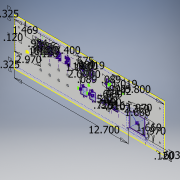
# Autodesk Inventor part: PDU_chassis
Saved by Autodesk Inventor 2017 (Build 210142000, 142)
## iProperties
Created: 2017-02-13
Part Number: PDU_chassis
Material: Generic
Document SubType Name: Modeling
Designer: Zara
Density: 1 g/cm^3
Appearance: Default
Author: Zara
Autodesk Inventor part; units mm, degrees
ref_plane "YZ Plane" through (0, 0, 0) normal (1, 0, 0) x (0, 1, 0)
ref_plane "XZ Plane" through (0, 0, 0) normal (0, 1, 0) x (-1, 0, 0)
ref_plane "XY Plane" through (0, 0, 0) normal (0, 0, 1) x (1, 0, 0)
sketch "Sketch1" plane through (0, 0, 0) normal (0, 0, 1) x (1, 0, 0)
  line L0 (-212.471, -66.294) -> (212.471, -66.294)
  line L1 (212.471, -66.294) -> (212.471, 66.294)
  line L2 (212.471, 66.294) -> (-212.471, 66.294)
  line L3 (-212.471, 66.294) -> (-212.471, -66.294)
  line L4 (-212.471, -66.294) -> (212.471, 66.294) construction
  line L5 (212.471, -66.294) -> (-212.471, 66.294) construction
  point P0 (0, 0)
  dimension "d0" = 424.942
  dimension "d1" = 132.588
  constraints: 12 end point, 2 midpoint, 2 parallel, 1 horizontal, 1 perpendicular
  measures "d0" distance of L1.end L2.end
  measures "d1" distance of L0.end L1.end
extrude "pdu" add sketch "Sketch1" along normal blind 1.651
sketch "dsub9 sketch" plane through (0, 0, 1.651) normal (0, 0, 1) x (1, 0, 0)
  line L0 (209.423, 58.039) -> (-209.423, 58.039) construction
  line L1 (-209.423, 58.039) -> (-209.423, -58.039) construction
  line L2 (-209.423, -58.039) -> (209.423, -58.039) construction
  line L3 (209.423, -58.039) -> (209.423, 58.039) construction
  line L4 (212.471, 66.294) -> (-212.471, 66.294) construction
  line L5 (-212.471, -66.294) -> (212.471, -66.294) construction
  line L6 (-212.471, 66.294) -> (-212.471, -66.294) construction
  line L7 (212.471, -66.294) -> (212.471, 66.294) construction
  arc A0 (-131.445, 36.9951) -> (-133.3231, 38.571) centre (-133.0452, 36.9951) ccw
  arc A1 (-133.3231, 19.3918) -> (-131.445, 20.9677) centre (-133.0452, 20.9677) ccw
  arc A2 (-142.621, 22.374) -> (-141.2987, 20.7981) centre (-141.0208, 22.374) ccw
  arc A3 (-141.2987, 37.1647) -> (-142.621, 35.5888) centre (-141.0208, 35.5888) ccw
  line L8 (-131.445, 36.9951) -> (-131.445, 20.9677)
  line L9 (-142.621, 35.5888) -> (-142.621, 22.374)
  line L10 (-141.2987, 37.1647) -> (-133.3231, 38.571)
  line L11 (-133.3231, 19.3918) -> (-141.2987, 20.7981)
  line L12 (-131.445, 28.9814) -> (-142.621, 28.9814) construction
  line L13 (-137.033, 41.4814) -> (-137.033, 16.4814) construction
  arc A4 (-117.221, 22.374) -> (-115.8987, 20.7981) centre (-115.6208, 22.374) ccw
  arc A5 (-107.9231, 19.3918) -> (-106.045, 20.9677) centre (-107.6452, 20.9677) ccw
  line L14 (-106.045, 28.9814) -> (-117.221, 28.9814) construction
  arc A6 (-115.8987, 37.1647) -> (-117.221, 35.5888) centre (-115.6208, 35.5888) ccw
  line L15 (-115.8987, 37.1647) -> (-107.9231, 38.571)
  line L16 (-106.045, 36.9951) -> (-106.045, 20.9677)
  arc A7 (-106.045, 36.9951) -> (-107.9231, 38.571) centre (-107.6452, 36.9951) ccw
  line L17 (-111.633, 41.4814) -> (-111.633, 16.4814) construction
  line L18 (-107.9231, 19.3918) -> (-115.8987, 20.7981)
  line L19 (-117.221, 35.5888) -> (-117.221, 22.374)
  arc A8 (-91.821, 22.374) -> (-90.4987, 20.7981) centre (-90.2208, 22.374) ccw
  arc A9 (-82.5231, 19.3918) -> (-80.645, 20.9677) centre (-82.2452, 20.9677) ccw
  line L20 (-80.645, 28.9814) -> (-91.821, 28.9814) construction
  arc A10 (-90.4987, 37.1647) -> (-91.821, 35.5888) centre (-90.2208, 35.5888) ccw
  line L21 (-90.4987, 37.1647) -> (-82.5231, 38.571)
  line L22 (-80.645, 36.9951) -> (-80.645, 20.9677)
  arc A11 (-80.645, 36.9951) -> (-82.5231, 38.571) centre (-82.2452, 36.9951) ccw
  line L23 (-86.233, 41.4814) -> (-86.233, 16.4814) construction
  line L24 (-82.5231, 19.3918) -> (-90.4987, 20.7981)
  line L25 (-91.821, 35.5888) -> (-91.821, 22.374)
  arc A12 (-66.421, 22.374) -> (-65.0987, 20.7981) centre (-64.8208, 22.374) ccw
  arc A13 (-57.1231, 19.3918) -> (-55.245, 20.9677) centre (-56.8452, 20.9677) ccw
  line L26 (-55.245, 28.9814) -> (-66.421, 28.9814) construction
  arc A14 (-65.0987, 37.1647) -> (-66.421, 35.5888) centre (-64.8208, 35.5888) ccw
  line L27 (-65.0987, 37.1647) -> (-57.1231, 38.571)
  line L28 (-55.245, 36.9951) -> (-55.245, 20.9677)
  arc A15 (-55.245, 36.9951) -> (-57.1231, 38.571) centre (-56.8452, 36.9951) ccw
  line L29 (-60.833, 41.4814) -> (-60.833, 16.4814) construction
  line L30 (-57.1231, 19.3918) -> (-65.0987, 20.7981)
  line L31 (-66.421, 35.5888) -> (-66.421, 22.374)
  line L32 (-133.3569, 38.565) -> (-128.9307, 40.2756) construction
  line L33 (-131.445, 32.3846) -> (-131.445, 46.6583) construction
  line L34 (-131.445, 25.0932) -> (-131.445, 19.1695) construction
  line L35 (-131.5619, 19.0813) -> (-130.7736, 22.0343) construction
  point P0 (0, 0)
  point P1 (-137.033, 28.9814)
  point P2 (-111.633, 28.9814)
  point P3 (-86.233, 28.9814)
  point P4 (-60.833, 28.9814)
  point P5 (-131.445, 19.5191)
  point P6 (-131.445, 39.3039)
  dimension "d24" = 38.1
  dimension "d13" = 8.255
  dimension "d14" = 8.255
  dimension "d15" = 3.048
  dimension "d16" = 3.048
  dimension "d381" = 3.2004
  dimension "d386" = 3.2004
  dimension "d391" = 3.2004
  dimension "d396" = 3.2004
  dimension "d397" = 16.0274
  dimension "d399" = 11.176
  dimension "d401" = 25
  dimension "d402" = 37.3126
  dimension "d403" = 75.438
  dimension "d406" = 25.4
  dimension "d420" = 100
  constraints: 64 end point, 32 point on circle, 16 centre point, 8 coincident, 8 point on line, 8 tangent, 5 vertical, 4 midpoint, 3 horizontal, 2 parallel, 2 perpendicular, 1 collinear, 86 other
  measures "d13" distance between parallel lines of L4 L0
  measures "d14" distance between parallel lines of L5 L2
  measures "d15" distance between parallel lines of L6 L1
  measures "d16" distance between parallel lines of L7 L3
  measures "d381" diameter of A0
  measures "d386" diameter of A1
  measures "d391" diameter of A2
  measures "d396" diameter of A3
  measures "d397" distance of A1.centre A0.centre
  measures "d399" distance between parallel lines of L9 L8
  measures "d401" distance of L13.start L13.end
  measures "d402" distance between parallel lines of L4 L12
  measures "d403" distance between parallel lines of L13 L6
  measures "d406" distance of A2.centre A4.centre
  measures "d420" angle of L11 L8
sketch "CAT7 sketch" plane through (0, 0, 1.651) normal (0, 0, 1) x (1, 0, 0)
  line L0 (-24.511, 40.4114) -> (-7.366, 40.4114)
  line L1 (-7.366, 40.4114) -> (-7.366, 17.5514)
  line L2 (-7.366, 17.5514) -> (-24.511, 17.5514)
  line L3 (-24.511, 17.5514) -> (-24.511, 40.4114)
  line L4 (-29.3489, 28.9814) -> (14.0188, 28.9814) construction
  circle A0 centre (-15.9385, 43.4848) radius 1.1303
  circle A1 centre (-15.9385, 14.478) radius 1.1303
  line L5 (-15.9385, 43.4848) -> (-15.9385, 14.478) construction
  line L6 (-212.471, -66.294) -> (212.471, -66.294) construction
  line L7 (-212.471, 66.294) -> (-212.471, -66.294) construction
  line L8 (32.9446, 29.4386) -> (89.0123, 29.4386) construction
  line L9 (48.006, 40.4114) -> (65.151, 40.4114)
  line L10 (65.151, 40.4114) -> (65.151, 17.5514)
  line L11 (65.151, 17.5514) -> (48.006, 17.5514)
  line L12 (48.006, 17.5514) -> (48.006, 40.4114)
  circle A2 centre (56.5785, 43.942) radius 1.1303
  circle A3 centre (56.5785, 14.9352) radius 1.1303
  line L13 (56.5785, 43.942) -> (56.5785, 14.9352) construction
  line L14 (212.471, 66.294) -> (-212.471, 66.294) projected
  line L15 (-212.471, -66.294) -> (212.471, -66.294) projected
  line L16 (212.471, -66.294) -> (212.471, 66.294) projected
  line L17 (212.471, 66.294) -> (-212.471, 66.294) projected
  line L18 (-212.471, 66.294) -> (-212.471, -66.294) projected
  line L19 (0.889, 40.4114) -> (18.034, 40.4114)
  line L20 (18.034, 40.4114) -> (18.034, 17.5514)
  line L21 (18.034, 17.5514) -> (0.889, 17.5514)
  line L22 (0.889, 17.5514) -> (0.889, 40.4114)
  line L23 (9.4615, 43.4848) -> (9.4615, 14.478) construction
  circle A4 centre (9.4615, 43.4848) radius 1.1303
  circle A5 centre (9.4615, 14.478) radius 1.1303
  line L24 (-24.511, -10.3886) -> (-7.366, -10.3886)
  line L25 (-7.366, -10.3886) -> (-7.366, -33.2486)
  line L26 (-7.366, -33.2486) -> (-24.511, -33.2486)
  line L27 (-24.511, -33.2486) -> (-24.511, -10.3886)
  line L28 (-15.9385, -7.3152) -> (-15.9385, -36.322) construction
  circle A6 centre (-15.9385, -7.3152) radius 1.1303
  circle A7 centre (-15.9385, -36.322) radius 1.1303
  line L29 (0.889, -10.3886) -> (18.034, -10.3886)
  line L30 (18.034, -10.3886) -> (18.034, -33.2486)
  line L31 (18.034, -33.2486) -> (0.889, -33.2486)
  line L32 (0.889, -33.2486) -> (0.889, -10.3886)
  line L33 (9.4615, -7.3152) -> (9.4615, -36.322) construction
  circle A8 centre (9.4615, -7.3152) radius 1.1303
  circle A9 centre (9.4615, -36.322) radius 1.1303
  line L34 (-15.9385, -21.8186) -> (111.9618, -21.8186) construction
  point P0 (-24.511, 28.9814)
  point P1 (-15.9385, 40.4114)
  point P2 (-15.9385, 28.9814)
  point P3 (48.006, 28.9814)
  point P4 (56.5785, 40.4114)
  point P5 (56.5785, 29.4386)
  point P6 (98.2853, 29.4386)
  point P7 (9.4615, 40.4114)
  point P8 (0.889, 28.9814)
  point P9 (-3.9489, 28.9814)
  point P10 (9.4615, 28.9814)
  point P11 (-15.9385, -10.3886)
  point P12 (-24.511, -21.8186)
  point P13 (-29.3489, -21.8186)
  point P14 (9.4615, -10.3886)
  point P15 (0.889, -21.8186)
  point P16 (-3.9489, -21.8186)
  point P17 (9.4615, -21.8186)
  dimension "d56" = 47.0408
  dimension "d47" = 22.86
  dimension "d49" = 2.2606
  dimension "d50" = 2.2606
  dimension "d51" = 29.0068
  dimension "d146" = 22.86
  dimension "d147" = 17.145
  dimension "d148" = 2.2606
  dimension "d149" = 2.2606
  dimension "d150" = 29.0068
  dimension "d152" = 25.8826
  dimension "d236" = 25.4
  dimension "d239" = 50.8
  dimension "d243" = 147.32
  dimension "d244" = 187.96
  dimension "d245" = 17.145
  dimension "d246" = 25.8826
  constraints: 56 end point, 10 centre point, 7 point on line, 6 midpoint, 5 horizontal, 4 parallel, 4 vertical, 2 collinear, 2 perpendicular, 49 other
  measures "d47" distance of L0.end L1.end
  measures "d49" diameter of A0
  measures "d50" diameter of A1
  measures "d51" distance of L5.end L5.start
  measures "d146" distance of L9.end L11.start
  measures "d147" distance of L11.start L12.start
  measures "d148" diameter of A2
  measures "d149" diameter of A3
  measures "d150" distance of L13.end L13.start
  measures "d152" distance between parallel lines of L14 L9
  measures "d236" distance of L0.start L19.start
  measures "d239" distance of L0.start L24.start
  measures "d243" distance between parallel lines of L16 L10
  measures "d244" distance between parallel lines of L3 L7
  measures "d245" distance of L0.start L0.end
  measures "d246" distance between parallel lines of L17 L0
sketch "airflow sketch" plane through (0, 0, 1.651) normal (0, 0, 1) x (1, 0, 0)
  line L0 (-212.471, -66.294) -> (212.471, -66.294) construction
  line L1 (110.109, -50.9778) -> (160.147, -50.9778) construction
  line L2 (160.147, -50.9778) -> (160.147, -0.9398) construction
  line L3 (160.147, -0.9398) -> (110.109, -0.9398) construction
  line L4 (110.109, -0.9398) -> (110.109, -50.9778) construction
  line L5 (110.109, -50.9778) -> (160.147, -0.9398) construction
  line L6 (160.147, -50.9778) -> (110.109, -0.9398) construction
  line L7 (-212.471, 66.294) -> (-212.471, -66.294) construction
  line L8 (114.046, -47.0408) -> (156.21, -47.0408)
  line L9 (156.21, -47.0408) -> (156.21, -4.8768)
  line L10 (156.21, -4.8768) -> (114.046, -4.8768)
  line L11 (114.046, -4.8768) -> (114.046, -47.0408)
  line L12 (114.046, -47.0408) -> (156.21, -4.8768) construction
  line L13 (156.21, -47.0408) -> (114.046, -4.8768) construction
  line L14 (105.156, -55.9308) -> (165.1, -55.9308) construction
  line L15 (165.1, -55.9308) -> (165.1, 4.0132) construction
  line L16 (165.1, 4.0132) -> (105.156, 4.0132) construction
  line L17 (105.156, 4.0132) -> (105.156, -55.9308) construction
  line L18 (105.156, -55.9308) -> (165.1, 4.0132) construction
  line L19 (165.1, -55.9308) -> (105.156, 4.0132) construction
  point P0 (0, 0)
  point P1 (0, 0)
  point P2 (135.128, -25.9588)
  point P3 (135.128, -25.9588)
  dimension "d221" = 322.58
  dimension "d222" = 15.3162
  dimension "d223" = 50.038
  dimension "d224" = 50.038
  dimension "d225" = 42.164
  dimension "d226" = 42.164
  dimension "d279" = 59.944
  constraints: 36 end point, 8 midpoint, 6 parallel, 4 coincident, 3 horizontal, 3 perpendicular, 1 point on line
  measures "d221" distance between parallel lines of L4 L7
  measures "d222" distance between parallel lines of L1 L0
  measures "d223" distance of L2.end L3.end
  measures "d224" distance of L1.end L2.end
  measures "d225" distance of L9.end L10.end
  measures "d226" distance of L8.end L9.end
  measures "d279" distance of L15.end L16.end
extrude "airflow cutout" cut sketch "airflow sketch" against normal through all
sketch "sma" plane through (0, 0, 1.651) normal (0, 0, 1) x (1, 0, 0)
  line L0 (-175.126, 2.9121) -> (-175.126, -16.382) construction
  line L1 (-183.1756, -6.2272) -> (-164.6712, -6.2272) construction
  arc A0 (-177.92, -7.7352) -> (-177.92, -4.7191) centre (-175.126, -6.2272) ccw
  line L2 (-177.92, -4.7191) -> (-177.92, -7.7352)
  line L3 (-137.033, 41.9354) -> (-137.033, 16.9418) construction
  line L4 (-137.026, 2.9121) -> (-137.026, -16.382) construction
  arc A1 (-139.82, -7.7352) -> (-139.82, -4.7191) centre (-137.026, -6.2272) ccw
  line L5 (-139.82, -4.7191) -> (-139.82, -7.7352)
  line L6 (-145.0756, -6.2272) -> (-126.5712, -6.2272) construction
  line L7 (-175.126, -22.4879) -> (-175.126, -41.782) construction
  arc A2 (-177.92, -33.1352) -> (-177.92, -30.1191) centre (-175.126, -31.6272) ccw
  line L8 (-177.92, -30.1191) -> (-177.92, -33.1352)
  line L9 (-183.1756, -31.6272) -> (-164.6712, -31.6272) construction
  line L10 (-137.026, -22.4879) -> (-137.026, -41.782) construction
  arc A3 (-139.82, -33.1352) -> (-139.82, -30.1191) centre (-137.026, -31.6272) ccw
  line L11 (-139.82, -30.1191) -> (-139.82, -33.1352)
  line L12 (-145.0756, -31.6272) -> (-126.5712, -31.6272) construction
  line L13 (-111.626, -22.4879) -> (-111.626, -41.782) construction
  line L14 (-114.42, -30.1191) -> (-114.42, -33.1352)
  arc A4 (-114.42, -33.1352) -> (-114.42, -30.1191) centre (-111.626, -31.6272) ccw
  line L15 (-114.42, -4.7191) -> (-114.42, -7.7352)
  line L16 (-119.6756, -31.6272) -> (-101.1712, -31.6272) construction
  arc A5 (-114.42, -7.7352) -> (-114.42, -4.7191) centre (-111.626, -6.2272) ccw
  line L17 (-119.6756, -6.2272) -> (-101.1712, -6.2272) construction
  line L18 (-86.226, -22.4879) -> (-86.226, -41.782) construction
  line L19 (-89.02, -30.1191) -> (-89.02, -33.1352)
  arc A6 (-89.02, -33.1352) -> (-89.02, -30.1191) centre (-86.226, -31.6272) ccw
  line L20 (-89.02, -4.7191) -> (-89.02, -7.7352)
  line L21 (-94.2756, -31.6272) -> (-75.7712, -31.6272) construction
  arc A7 (-89.02, -7.7352) -> (-89.02, -4.7191) centre (-86.226, -6.2272) ccw
  line L22 (-94.2756, -6.2272) -> (-75.7712, -6.2272) construction
  line L23 (-60.826, -22.4879) -> (-60.826, -41.782) construction
  line L24 (-63.62, -30.1191) -> (-63.62, -33.1352)
  arc A8 (-63.62, -33.1352) -> (-63.62, -30.1191) centre (-60.826, -31.6272) ccw
  line L25 (-63.62, -4.7191) -> (-63.62, -7.7352)
  line L26 (-68.8756, -31.6272) -> (-50.3712, -31.6272) construction
  arc A9 (-63.62, -7.7352) -> (-63.62, -4.7191) centre (-60.826, -6.2272) ccw
  line L27 (-68.8756, -6.2272) -> (-50.3712, -6.2272) construction
  point P0 (0, 0)
  point P1 (-171.951, -6.2272)
  point P2 (-133.851, -6.2272)
  point P3 (-171.951, -31.6272)
  point P4 (-133.851, -31.6272)
  point P5 (-108.451, -31.6272)
  point P6 (-111.626, -16.382)
  point P7 (-108.451, -6.2272)
  point P8 (-83.051, -31.6272)
  point P9 (-86.226, -16.382)
  point P10 (-83.051, -6.2272)
  point P11 (-57.651, -31.6272)
  point P12 (-60.826, -16.382)
  point P13 (-57.651, -6.2272)
  dimension "d123" = 6.35
  dimension "d124" = 5.969
  dimension "d191" = 38.1
  dimension "d198" = 25.4
  dimension "d205" = 25.4
  constraints: 54 end point, 30 point on circle, 27 point on line, 10 centre point, 3 collinear, 3 horizontal, 3 vertical, 99 other
  measures "d123" diameter of A0
  measures "d124" distance from line of point (-171.951, -6.227) L2
  measures "d191" distance of L0.start L4.start
  measures "d198" distance of L0.start L7.start
  measures "d205" distance of L12.start L16.start
extrude "sma cutouts" cut sketch "sma" against normal through all
sketch "lc and sc" plane through (0, 0, 1.651) normal (0, 0, 1) x (1, 0, 0)
  arc A0 (-177.92, -7.7352) -> (-177.92, -4.7191) centre (-175.126, -6.2272) ccw projected
  line L0 (-177.92, -7.7352) -> (-177.92, -4.7191) projected
  line L1 (-212.471, -66.294) -> (212.471, -66.294) projected
  line L2 (212.471, -66.294) -> (212.471, 66.294) projected
  line L3 (212.471, 66.294) -> (-212.471, 66.294) projected
  line L4 (-212.471, 66.294) -> (-212.471, -66.294) projected
  line L5 (56.5785, 43.942) -> (56.5785, 14.9352) construction
  line L6 (48.006, 40.4114) -> (65.151, 40.4114) projected
  line L7 (48.006, 17.5514) -> (48.006, 40.4114) projected
  line L8 (65.151, 17.5514) -> (48.006, 17.5514) projected
  line L9 (65.151, 40.4114) -> (65.151, 17.5514) projected
  circle A1 centre (56.5785, 14.9352) radius 1.1303 projected
  line L10 (-15.9385, -21.8186) -> (111.9618, -21.8186) construction
  line L11 (33.4137, -17.0688) -> (46.4185, -17.0688)
  line L12 (46.4185, -17.0688) -> (46.4185, -26.5684)
  line L13 (46.4185, -26.5684) -> (33.4137, -26.5684)
  line L14 (33.4137, -26.5684) -> (33.4137, -17.0688)
  line L15 (33.4137, -17.0688) -> (46.4185, -26.5684) construction
  line L16 (46.4185, -17.0688) -> (33.4137, -26.5684) construction
  line L17 (30.8991, -21.8186) -> (48.9331, -21.8186) construction
  line L18 (39.9161, -21.8186) -> (39.9161, -14.0945) construction
  line L19 (18.034, -10.3886) -> (18.034, -33.2486) projected
  line L20 (56.5785, 14.9352) -> (56.5785, -41.5551) construction
  line L21 (66.7385, -26.6446) -> (79.8449, -26.6446)
  line L22 (79.8449, -26.6446) -> (79.8449, -16.9926)
  line L23 (79.8449, -16.9926) -> (66.7385, -16.9926)
  line L24 (66.7385, -16.9926) -> (66.7385, -26.6446)
  line L25 (66.7385, -26.6446) -> (79.8449, -16.9926) construction
  line L26 (79.8449, -26.6446) -> (66.7385, -16.9926) construction
  line L27 (64.2747, -21.8186) -> (82.3087, -21.8186) construction
  line L28 (73.2917, -16.3932) -> (73.2917, -27.244) construction
  point P0 (0, 0)
  point P1 (39.9161, -21.8186)
  point P2 (39.9161, -21.8186)
  point P3 (73.2917, -21.8186)
  point P4 (73.2917, -21.8186)
  point P5 (73.2917, -21.8186)
  dimension "d247" = 13.0048
  dimension "d248" = 9.4996
  dimension "d249" = 18.034
  dimension "d262" = 10.16
  dimension "d263" = 18.034
  dimension "d264" = 13.1064
  dimension "d265" = 9.652
  dimension "d266" = 10.16
  constraints: 34 end point, 11 midpoint, 4 coincident, 4 horizontal, 4 parallel, 3 point on line, 2 perpendicular, 2 vertical
  measures "d247" distance of L14.end L12.start
  measures "d248" distance of L12.start L12.end
  measures "d249" distance of L17.start L17.end
  measures "d262" distance between parallel lines of L20 L12
  measures "d263" distance of L27.start L27.end
  measures "d264" distance of L22.end L23.end
  measures "d265" distance of L21.end L22.end
  measures "d266" distance between parallel lines of L20 L24
hole "lc hole" at (48.9331, -21.8186, 1.651) at (30.8991, -21.8186, 1.651) direction (0, 0, -1) diameter 2.3876 end through all clearance for "Countersunk Flat Head Screw ISO 2009/7046" size "M2" standard "ISO"
hole "airflow holes" at (160.147, -0.9398, 1.651) at (110.109, -0.9398, 1.651) at (110.109, -50.9778, 1.651) at (160.147, -50.9778, 1.651) direction (0, 0, -1) diameter 5.1054 end through all
extrude "Extrusion13" cut sketch "CAT7 sketch" against normal blind 25.4 contours L0 L1 L2 L3 | L9 L10 L11 L12 | L19 L20 L21 L22 | L24 L25 L26 L27 | L29 L30 L31 L32
hole "Hole8" at (-15.9385, 43.4848, 1.651) at (-15.9385, 14.478, 1.651) at (9.4615, 43.4848, 1.651) at (9.4615, 14.478, 1.651) at (-15.9385, -7.3152, 1.651) at (-15.9385, -36.322, 1.651) at (9.4615, -7.3152, 1.651) at (9.4615, -36.322, 1.651) at (56.5785, 14.9352, 1.651) at (56.5785, 43.942, 1.651) direction (0, 0, -1) diameter 3.2766 end through all
extrude "Extrusion14" cut sketch "lc and sc" against normal blind 25.4 contours L11 L12 L13 L14 | L24 L23 L22 L21
hole "sc hole" at (82.3087, -21.8186, 1.651) at (64.2747, -21.8186, 1.651) direction (0, 0, -1) diameter 2.4384 end through all clearance for "Flat Head Machine Screw (82)" size "#2" standard "Ansi Unified Screw Threads"
fillet "lc fillets" radius 0.508 4 edges at (33.4137, -26.5684, 0.8255) (46.4185, -17.0688, 0.8255) (46.4185, -26.5684, 0.8255) (33.4137, -17.0688, 0.8255)
fillet "sc fillets" radius 0.508 4 edges at (66.7385, -16.9926, 0.8255) (66.7385, -26.6446, 0.8255) (79.8449, -16.9926, 0.8255) (79.8449, -26.6446, 0.8255)
sketch "brackets" plane through (0, 0, 1.651) normal (0, 0, 1) x (1, 0, 0)
  line L0 (-212.471, 66.294) -> (-212.471, -66.294) construction
  line L1 (-212.471, 54.61) -> (-193.421, 54.61) construction
  line L2 (-193.421, 54.61) -> (-193.421, -54.61) construction
  line L3 (-193.421, -54.61) -> (-212.471, -54.61) construction
  line L4 (-212.471, -54.61) -> (-212.471, 54.61) construction
  line L5 (212.471, 66.294) -> (-212.471, 66.294) construction
  line L6 (212.471, -66.294) -> (212.471, 66.294) construction
  line L7 (212.471, 54.61) -> (193.421, 54.61) construction
  line L8 (193.421, 54.61) -> (193.421, -54.61) construction
  line L9 (193.421, -54.61) -> (212.471, -54.61) construction
  line L10 (212.471, -54.61) -> (212.471, 54.61) construction
  point P0 (0, 0)
  point P1 (199.4154, 41.91)
  point P2 (199.4154, -41.91)
  point P3 (-199.4154, 41.91)
  point P4 (-199.4154, -41.91)
  dimension "d280" = 19.05
  dimension "d281" = 109.22
  dimension "d282" = 11.684
  dimension "d286" = 19.05
  dimension "d287" = 109.22
  dimension "d288" = 11.684
  dimension "d291" = 12.7
  dimension "d292" = 12.7
  dimension "d293" = 12.7
  dimension "d295" = 12.7
  dimension "d297" = 5.9944
  dimension "d298" = 5.9944
  dimension "d306" = 5.9944
  dimension "d307" = 5.9944
  constraints: 16 end point, 4 parallel, 2 horizontal, 2 perpendicular, 2 point on line
  measures "d280" distance of L1.start L1.end
  measures "d281" distance of L1.end L2.end
  measures "d282" distance between parallel lines of L5 L1
  measures "d286" distance of L7.start L7.end
  measures "d287" distance of L7.end L8.end
  measures "d288" distance between parallel lines of L5 L7
  measures "d291" distance from line of point (199.415, -41.91) L9
  measures "d292" distance from line of point (199.415, 41.91) L7
  measures "d293" distance from line of point (-199.415, 41.91) L1
  measures "d295" distance from line of L3 point (-199.415, -41.91)
  measures "d297" distance from line of point (-199.415, 41.91) L2
  measures "d298" distance from line of point (-199.415, -41.91) L2
  measures "d306" distance from line of L8 point (199.415, -41.91)
  measures "d307" distance from line of L8 point (199.415, 41.91)
hole "Hole13" at (-199.4154, 41.91, 1.651) at (-199.4154, -41.91, 1.651) at (199.4154, 41.91, 1.651) at (199.4154, -41.91, 1.651) direction (0, 0, -1) diameter 4.2926 end through all
extrude "Extrusion16" cut sketch "dsub9 sketch" against normal through all
hole "Hole14" at (-137.033, 41.4814, 1.651) at (-137.033, 16.4814, 1.651) at (-111.633, 41.4814, 1.651) at (-111.633, 16.4814, 1.651) at (-86.233, 41.4814, 1.651) at (-86.233, 16.4814, 1.651) at (-60.833, 41.4814, 1.651) at (-60.833, 16.4814, 1.651) direction (0, 0, -1) diameter 2.9464 end through all
body "Solid1"
